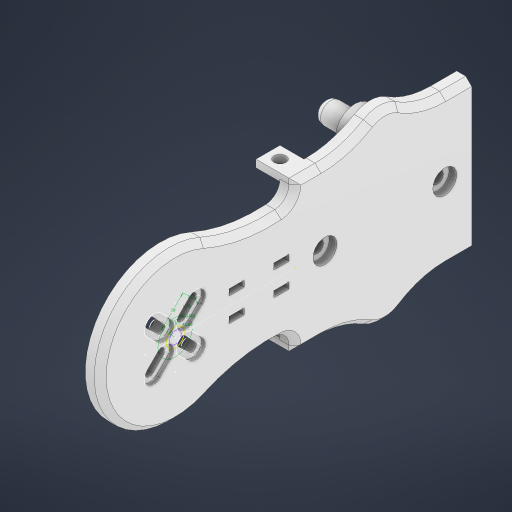
# Autodesk Inventor part: bldc_arm
Saved by Autodesk Inventor 2024.2 (Build 282272000, 272)
## iProperties
Created: 2024-03-15
Part Number: bldc_arm
Material: ABS Plastic
Document SubType Name: Modeling
Designer: jerem
Density: 1.06 g/cm^3
Appearance: Smooth - White
Mass: 32.0643 g
Surface Area: 145.548 cm^2
Volume: 30.2494 cm^3
Author: jerem
## iProperties of the stored document bldc_arm_3DPrint.ipt
Created: 2024-03-22
Part Number: bldc_arm_3DPrint
Material: Generic
Document SubType Name: Modeling
Designer: jerem
Density: 1 g/cm^3
Appearance: Default
Author: jerem
Autodesk Inventor part; units mm, degrees
ref_plane "YZ Plane" through (0, 0, 0) normal (1, 0, 0) x (0, 1, 0)
ref_plane "XZ Plane" through (0, 0, 0) normal (0, 1, 0) x (-1, 0, 0)
ref_plane "XY Plane" through (0, 0, 0) normal (0, 0, 1) x (1, 0, 0)
sketch "Sketch1" plane through (0, 0, 0) normal (1, 0, 0) x (0, 1, 0)
  line L0 (0, 0) -> (0, -10) construction
  line L1 (0, -10) -> (0, -50) construction
  circle A0 centre (0, -10) radius 2
  circle A1 centre (0, -50) radius 2
  line L2 (10, 0) -> (10, -59)
  line L3 (10, -59) -> (0, -59)
  line L4 (0, -59) -> (-10, -59)
  line L5 (-10, -59) -> (-10, 0)
  line L6 (0, 0) -> (10, 0)
  line L7 (0, 0) -> (-10, 0)
  line L8 (0, -50) -> (0, -59) construction
  circle A2 centre (0, 40) radius 25
  line L9 (10, 0) -> (10, 10)
  line L10 (10, 10) -> (-10, 10)
  line L11 (-10, 10) -> (-10, 0)
  arc A3 (22.8049, 29.7561) -> (10, -30) centre (155.8333, -30) ccw
  arc A4 (-10, -30) -> (-22.8049, 29.7561) centre (-155.8333, -30) ccw
  circle A5 centre (6.2862, 46.2862) radius 1.5
  circle A6 centre (5.3882, 34.6118) radius 1.5
  line L12 (0, -30) -> (21, -30) construction
  line L13 (0, -30) -> (-21, -30) construction
  circle A7 centre (21, -30) radius 3.5
  circle A8 centre (-21, -30) radius 3.5
  circle A9 centre (21, -30) radius 10
  circle A10 centre (-21, -30) radius 10
  circle A11 centre (21, -30) radius 6.5
  circle A12 centre (-21, -30) radius 6.5
  line L14 (-10, -59) -> (-25, -59)
  line L15 (10, -59) -> (25, -59)
  arc A13 (-28.9586, -23.9452) -> (-22.8049, 29.7561) centre (-71.0556, 8.082) ccw
  arc A14 (22.8049, 29.7561) -> (28.9586, -23.9452) centre (71.0556, 8.082) ccw
  line L16 (0, 0) -> (15, 0)
  line L17 (10, 0) -> (25, 0)
  line L18 (25, -59) -> (25, -50.3)
  arc A15 (29.3932, -35.4364) -> (25, -50.3) centre (52.3408, -50.3) ccw
  line L19 (25, 0) -> (25, -8.7)
  arc A16 (25, -8.7) -> (29.5297, -24.7804) centre (55.8075, -8.7) ccw
  line L20 (-10, 0) -> (-25, 0)
  line L21 (-25, -59) -> (-25, -50.3)
  arc A17 (-25, -50.3) -> (-29.3932, -35.4364) centre (-52.3408, -50.3) ccw
  line L22 (-25, 0) -> (-25, -8.7)
  arc A18 (-29.5297, -24.7804) -> (-25, -8.7) centre (-55.8075, -8.7) ccw
  line L23 (0, 40) -> (5.3882, 34.6118) construction
  line L24 (0, 40) -> (6.2862, 46.2862) construction
  line L25 (0, 40) -> (8.89, 40) construction
  line L26 (0, 40) -> (-5.3882, 45.3882) construction
  circle A19 centre (-5.3882, 45.3882) radius 1.5
  circle A20 centre (-6.2862, 33.7138) radius 1.5
  line L27 (0, 40) -> (-6.2862, 33.7138) construction
  circle A21 centre (5.3882, 34.6118) radius 3
  circle A22 centre (6.2862, 46.2862) radius 3
  circle A23 centre (-6.2862, 33.7138) radius 3
  circle A24 centre (-5.3882, 45.3882) radius 3
  circle A25 centre (0, -50) radius 4
  circle A26 centre (0, -10) radius 4
  circle A27 centre (0, 40) radius 3
  line L28 (7.3468, 45.2255) -> (2.6941, 41.3198)
  point P0 (-10, -30)
  point P1 (10, -30)
  point P2 (23.8246, -39.5928)
  point P3 (10, -63.336)
  point P4 (-30.2308, -33.8462)
  point P5 (28.9586, -23.9452)
  point P6 (22.8049, 29.7561)
  point P7 (30.2308, -26.1538)
  point P8 (18.7815, 0)
  point P9 (-18.7815, 0)
  point P10 (-13.1191, 0)
  point P11 (-29.3932, -35.4364)
  dimension "d18" = 3
  dimension "d138" = 6
  dimension "d0" = 4
  dimension "d1" = 4
  dimension "d2" = 40
  dimension "d3" = 10
  dimension "d5" = 9
  dimension "d7" = 10
  dimension "d8" = 10
  dimension "d9" = 50
  dimension "d12" = 30
  dimension "d13" = 10
  dimension "d14" = 20
  dimension "d19" = 3
  dimension "d30" = 21
  dimension "d31" = 7
  dimension "d32" = 7
  dimension "d33" = 20
  dimension "d34" = 20
  dimension "d38" = 3
  dimension "d48" = 15
  dimension "d55" = 15
  dimension "d56" = 8.7
  dimension "d57" = 8.7
  dimension "d58" = 15
  dimension "d91" = 7.62
  dimension "d93" = 8.89
  dimension "d95" = -45
  dimension "d96" = 6
  dimension "d97" = 6
  dimension "d98" = 6
  dimension "d99" = 6
  dimension "d134" = 8
  dimension "d135" = 8
  constraints: 59 end point, 26 centre point, 25 point on circle, 18 symmetric about line, 16 coincident, 8 point on line, 8 tangent, 7 perpendicular, 6 horizontal, 5 equal length, 5 vertical, 1 midpoint, 13 other
  measures "d0" diameter of A0
  measures "d1" diameter of A1
  measures "d2" distance of L0.end L1.end
  measures "d3" distance of L0.start L0.end
  measures "d5" distance of L3.end L1.end
  measures "d7" distance from line of L12.start L5
  measures "d8" distance between parallel lines of L1 L2
  measures "d9" diameter of A2
  measures "d12" distance from line of L23.start L10
  measures "d13" distance of L2.start L9.end
  measures "d14" vertical distance of L0.end A3.end
  measures "d19" diameter of A6
  measures "d30" distance of L12.start L12.end
  measures "d31" diameter of A7
  measures "d32" diameter of A8
  measures "d33" diameter of A9
  measures "d34" diameter of A10
  measures "d38" radial gap between concentric circles of A11 A7
  measures "d48" distance of L4.end L14.end
  measures "d55" distance of L2.start L17.end
  measures "d56" distance of L15.end L18.end
  measures "d57" distance of L17.end L19.end
  measures "d58" distance of L2.end L15.end
  measures "d91" distance of L23.start L23.end
  measures "d93" distance of L23.start L24.end
  measures "d95" angle of L25 L23
  measures "d96" diameter of A21
  measures "d97" diameter of A22
  measures "d98" diameter of A23
  measures "d99" diameter of A24
  measures "d134" diameter of A25
  measures "d135" diameter of A26
extrude "Extrusion1" add sketch "Sketch1" along normal blind 5 contours L16 A3 L2 | L2 L3 L4 L5 L7 L6 | L6 L7 L11 L10 L9 | L9 L10 L11 L20 A4 A2 A3 L16 | A3 L16 L17 A14 A9 A15 L18 L15 L2 | A3 A14 L17 L16 | L5 A4 L20 | A2 | L5 L14 L21 A17 A10 A13 L20 A4 | L20 A13 A4 | L17 L19 A16 A9 A14 | A13 A10 A18 L22 L20 | A9 | A10 | L28 A5 | A5 L28 | A6 | A7 | A8 | A11 | A12 | A19 | A20 | A21 | A22 | A23 | A24 | A25 | A26 | A27
extrude "Extrusion3" add sketch "Sketch1" against normal blind 15 contours A7 | A8
extrude "Extrusion4" add sketch "Sketch1" against normal blind 5 contours A11 | A12
fillet "Face Fillet1" radius 5 1 edges at (2.5, -18.7815, 0)
fillet "Face Fillet2" radius 5 1 edges at (2.5, 18.7815, 0)
sketch "Sketch8" plane through (0, 0, 0) normal (-1, 0, 0) x (0, 0, 1)
  line L0 (0, 0) -> (0, -3)
  line L1 (30, -3) -> (30, 3)
  line L2 (30, 3) -> (0, 3)
  line L3 (0, 0) -> (0, 3)
  line L4 (30, -3) -> (0, -3)
  dimension "d102" = 3
  dimension "d104" = 6
  dimension "d105" = 30
  dimension "d121" = 6
  constraints: 10 end point, 2 vertical, 1 coincident, 1 collinear
  measures "d102" distance of L0.start L0.end
  measures "d104" distance of L1.start L1.end
  measures "d105" distance of L1.start L0.end
  measures "d121" distance between parallel lines of L4 L2
extrude "Extrusion9" cut sketch "Sketch8" against normal blind 2
fillet "Fillet2" radius 2 2 edges at (2, -3, 15) (2, 3, 15)
sketch "Sketch9" plane through (0, 0, 0) normal (-1, 0, 0) x (0, 0, 1)
  line L0 (7, -5) -> (2, -5)
  line L1 (2, -5) -> (2, -3)
  line L2 (2, -3) -> (7, -3)
  line L3 (7, -3) -> (7, -5)
  line L4 (0, 0) -> (3.7115, 0) construction
  line L5 (7, 5) -> (2, 5)
  line L6 (2, 5) -> (2, 3)
  line L7 (2, 3) -> (7, 3)
  line L8 (7, 3) -> (7, 5)
  line L9 (8.9306, 0) -> (12.6421, 0) construction
  line L10 (22, -5) -> (17, -5)
  line L11 (17, -5) -> (17, -3)
  line L12 (17, -3) -> (22, -3)
  line L13 (22, -3) -> (22, -5)
  line L14 (15, 0) -> (12.4386, 0) construction
  line L15 (22, 5) -> (17, 5)
  line L16 (17, 5) -> (17, 3)
  line L17 (17, 3) -> (22, 3)
  line L18 (22, 3) -> (22, 5)
  line L19 (17.6578, 0) -> (21.3692, 0) construction
  point P0 (0, 3)
  point P1 (8.7271, 3)
  dimension "d115" = 5
  dimension "d129" = 2
  dimension "d130" = 3
  dimension "d132" = 2
  dimension "d180" = 5
  dimension "d181" = 2
  dimension "d182" = 3
  dimension "d183" = 2
  dimension "d184" = 10
  constraints: 40 end point, 8 symmetric about line, 6 horizontal, 4 parallel, 3 collinear, 2 perpendicular, 2 point on line
  measures "d115" distance of L0.start L0.end
  measures "d129" distance of L2.end L0.start
  measures "d130" distance between parallel lines of L4 L2
  measures "d132" distance from line of L1 L4.start
  measures "d180" distance of L10.start L10.end
  measures "d181" distance of L12.end L10.start
  measures "d182" distance between parallel lines of L14 L12
  measures "d183" distance from line of L11 L14.start
  measures "d184" distance between parallel lines of L8 L16
extrude "Extrusion10" cut sketch "Sketch9" against normal up to surface (5 mm away)
extrude "Extrusion11" cut sketch "Sketch1" against normal blind 2.5 from surface at 5 contours A25 | A26
extrude "Extrusion12" cut sketch "Sketch1" along normal blind 3 contours A27
sketch "Sketch10" plane through (0, 0, 0) normal (-1, 0, 0) x (0, 0, 1)
  line L0 (-8.7, 25) -> (0, 25) projected
  line L1 (0, 25) -> (-8, 25)
  line L2 (-8, 25) -> (-8, 22.5)
  line L3 (-8, 22.5) -> (0, 22.5)
  line L4 (0, 22.5) -> (0, 25)
  point P0 (0, 0)
  dimension "d150" = 8
  dimension "d151" = 2.5
  constraints: 8 end point, 2 parallel, 1 horizontal, 1 perpendicular
  measures "d150" distance of L3.end L2.end
  measures "d151" distance of L2.end L1.end
extrude "Extrusion13" add sketch "Sketch10" along normal blind 8
sketch "Sketch12" plane through (0, 25, -8.7) normal (0, 1, 0) x (1, 0, 0)
  circle A0 centre (-4, -4.7) radius 2
  line L0 (-8, -8.7) -> (5, -8.7) projected
  line L1 (-8, -8.7) -> (-8, -0.7) projected
  point P0 (0, -8.7)
  dimension "d152" = 4
  dimension "d153" = 4
  dimension "d154" = 4
  constraints: 1 centre point
  measures "d152" diameter of A0
  measures "d153" distance from line of L0 A0.centre
  measures "d154" distance from line of L1 A0.centre
extrude "Extrusion15" cut sketch "Sketch12" against normal up to surface (2.5 mm away)
mirror "Mirror1" about plane through (0, 0, 0) normal (0, 1, 0) of "Extrusion13", "Extrusion15"
fillet "Fillet4" radius 2 2 edges at (-15, -24.5, -30) (-15, 17.5, -30)
chamfer "Chamfer2" distance 2 angle 45 17 edges at (5, 0, 65) (5, -19.0046, 17.4944) (5, -19.8398, 1.3525) (5, -24.1298, 0) (5, 19.0046, 17.4944) (5, 19.8398, 1.3525) (5, 24.1298, 0) (5, 26.154, -17.0531) (5, 25, -4.35) (5, 30.9992, -30.1281) (5, 26.1213, -42.5504) (5, 25, -54.65) (5, -26.154, -17.0531) (5, -30.9992, -30.1281) (5, -26.1213, -42.5504) (5, -25, -54.65) (5, -25, -4.35)
sketch "Sketch13" plane through (5, 0, 0) normal (1, 0, 0) x (0, 0, -1)
  point P0 (0, 0)
sketch "Sketch14" plane through (5, 0, 0) normal (1, 0, 0) x (0, 0, -1)
  circle A0 centre (-40, 0) radius 3 projected
  line L0 (-40, 0) -> (0, 0) construction
  line L1 (-40, 0) -> (-32.9289, 7.0711) construction
  line L2 (-40, 0) -> (-30, 0) construction
  arc A1 (-31.8683, 6.0104) -> (-33.9896, 8.1317) centre (-32.9289, 7.0711) ccw
  arc A2 (-37.5251, 4.5962) -> (-35.4038, 2.4749) centre (-36.4645, 3.5355) ccw
  line L3 (-37.5251, 4.5962) -> (-33.9896, 8.1317)
  line L4 (-31.8683, 6.0104) -> (-35.4038, 2.4749)
  circle A3 centre (-40, 0) radius 2.0021
  line L5 (-35.227, 9.3692) -> (-38.7626, 5.8336)
  arc A4 (-38.7626, 5.8336) -> (-34.1664, 1.2374) centre (-36.4645, 3.5355) ccw
  line L6 (-34.1664, 1.2374) -> (-30.6308, 4.773)
  arc A5 (-30.6308, 4.773) -> (-35.227, 9.3692) centre (-32.9289, 7.0711) ccw
  arc A6 (-44.5962, 2.4749) -> (-42.4749, 4.5962) centre (-43.5355, 3.5355) ccw
  arc A7 (-45.8336, 1.2374) -> (-41.2374, 5.8336) centre (-43.5355, 3.5355) ccw
  line L7 (-46.0104, 8.1317) -> (-42.4749, 4.5962)
  arc A8 (-44.773, 9.3692) -> (-49.3692, 4.773) centre (-47.0711, 7.0711) ccw
  arc A9 (-46.0104, 8.1317) -> (-48.1317, 6.0104) centre (-47.0711, 7.0711) ccw
  line L8 (-44.5962, 2.4749) -> (-48.1317, 6.0104)
  line L9 (-49.3692, 4.773) -> (-45.8336, 1.2374)
  line L10 (-41.2374, 5.8336) -> (-44.773, 9.3692)
  arc A10 (-42.4749, -4.5962) -> (-44.5962, -2.4749) centre (-43.5355, -3.5355) ccw
  arc A11 (-41.2374, -5.8336) -> (-45.8336, -1.2374) centre (-43.5355, -3.5355) ccw
  line L11 (-48.1317, -6.0104) -> (-44.5962, -2.4749)
  arc A12 (-49.3692, -4.773) -> (-44.773, -9.3692) centre (-47.0711, -7.0711) ccw
  arc A13 (-48.1317, -6.0104) -> (-46.0104, -8.1317) centre (-47.0711, -7.0711) ccw
  line L12 (-42.4749, -4.5962) -> (-46.0104, -8.1317)
  line L13 (-44.773, -9.3692) -> (-41.2374, -5.8336)
  line L14 (-45.8336, -1.2374) -> (-49.3692, -4.773)
  arc A14 (-35.4038, -2.4749) -> (-37.5251, -4.5962) centre (-36.4645, -3.5355) ccw
  arc A15 (-34.1664, -1.2374) -> (-38.7626, -5.8336) centre (-36.4645, -3.5355) ccw
  line L15 (-33.9896, -8.1317) -> (-37.5251, -4.5962)
  arc A16 (-35.227, -9.3692) -> (-30.6308, -4.773) centre (-32.9289, -7.0711) ccw
  arc A17 (-33.9896, -8.1317) -> (-31.8683, -6.0104) centre (-32.9289, -7.0711) ccw
  line L16 (-35.4038, -2.4749) -> (-31.8683, -6.0104)
  line L17 (-30.6308, -4.773) -> (-34.1664, -1.2374)
  line L18 (-38.7626, -5.8336) -> (-35.227, -9.3692)
  point P0 (-40, 10)
  point P1 (-50, 0)
  point P2 (-40, -10)
  dimension "d161" = 45
  dimension "d162" = 3
  dimension "d163" = 3
  dimension "d164" = 10
  dimension "d165" = 5
  dimension "d166" = 1.75
  dimension "d169" = 360
  constraints: 38 end point, 32 point on circle, 17 centre point, 10 coincident, 2 horizontal, 2 parallel, 2 tangent, 1 equal length, 1 midpoint, 90 other
  measures "d161" angle of L2 L1
  measures "d162" diameter of A1
  measures "d163" diameter of A2
  measures "d164" distance of L0.start L1.end
  measures "d165" distance of L0.start A2.centre
  measures "d166" distance between parallel lines of L3 L5
extrude "Extrusion16" cut sketch "Sketch14" against normal up to surface (5 mm away) contours L4 A2 L3 A1 | L8 A9 L7 A6 | L12 A13 L11 A10 | L16 A17 L15 A14
extrude "Extrusion17" cut sketch "Sketch14" against normal blind 1.5 contours A4 A3 A0 | A0 A4 L5 A5 L6 | A15 L17 A16 L18 A0 | A0 A15 A3 | A4 A3 | A3 A15 | A7 A3 A0 | A0 A7 L9 A8 L10 | A11 L13 A12 L14 A0 | A0 A11 A3 | A7 A3 | A3 A11
fillet "Fillet5" radius 3 1 edges at (3, -3, 40)
sketch "Sketch15" plane through (0, 0, 0) normal (-1, 0, 0) x (0, 0, 1)
  line L0 (0, -3) -> (-5, -3)
  line L1 (-5, -3) -> (-5, 3)
  line L2 (-5, 3) -> (0, 3)
  line L3 (0, 1) -> (0, 3) projected
  line L4 (0, -3) -> (0, 3)
  point P0 (0, 0)
  dimension "d176" = 5
  constraints: 8 end point, 2 coincident, 2 perpendicular, 1 horizontal, 1 vertical
  measures "d176" distance of L0.start L0.end
extrude "Extrusion18" cut sketch "Sketch15" against normal up to surface (2 mm away)
fillet "Fillet6" radius 2 2 edges at (2, -3, -2.5) (2, 3, -2.5)
equation "\"d18\" = M3_HOLE_D"
equation "\"d0\" = M4_HOLE_D"
equation "\"d1\" = d0"
equation "\"d14\" = 0.5 * d2"
equation "\"d19\" = d18"
equation "\"d32\" = d31"
equation "\"d34\" = d33"
equation "\"M4_HOLE_D\" = 4"
equation "\"M3_HOLE_D\" = 3"
equation "\"d88\" = 3"
body "Solid1"
